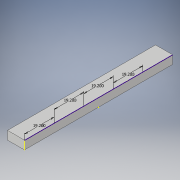
# Autodesk Inventor part: mars rover landscape part 2
Saved by Autodesk Inventor 2017 (Build 210142000, 142)
## iProperties
Created: 2017-09-13
Part Number: mars rover landscape part 2
Material: Generic
Document SubType Name: Modeling
Designer: 602199
Density: 1 g/cm^3
Appearance: Default
Author: 602199
Autodesk Inventor part; units mm, degrees
ref_plane "YZ Plane" through (0, 0, 0) normal (1, 0, 0) x (0, 1, 0)
ref_plane "XZ Plane" through (0, 0, 0) normal (0, 1, 0) x (-1, 0, 0)
ref_plane "XY Plane" through (0, 0, 0) normal (0, 0, 1) x (1, 0, 0)
sketch "Sketch1" plane through (0, 0, 0) normal (0, 1, 0) x (-1, 0, 0)
  line L0 (-139.7, 1219.2) -> (139.7, 1219.2)
  line L1 (139.7, 1219.2) -> (139.7, -1219.2)
  line L2 (139.7, -1219.2) -> (-139.7, -1219.2)
  line L3 (-139.7, -1219.2) -> (-139.7, 1219.2)
  line L4 (-139.7, 1219.2) -> (139.7, -1219.2) construction
  line L5 (139.7, 1219.2) -> (-139.7, -1219.2) construction
  point P0 (0, 0)
  dimension "d0" = 279.4
  dimension "d1" = 2438.4
  constraints: 12 end point, 2 midpoint, 2 parallel, 1 horizontal, 1 perpendicular
  measures "d0" distance of L1.end L2.end
  measures "d1" distance of L0.end L1.end
extrude "Extrusion1" add sketch "Sketch1" along normal blind 139.7
sketch "Sketch2" plane through (139.7, 0, 1219.2) normal (1, 0, 0) x (0, 0, -1)
  line L0 (0, 0) -> (0, 139.7) projected
  line L1 (0, 139.7) -> (487.68, 139.7)
  line L2 (0, 139.7) -> (2438.4, 139.7) projected
  line L3 (487.68, 139.7) -> (975.36, 139.7)
  line L4 (975.36, 139.7) -> (1463.04, 139.7)
  line L5 (1463.04, 139.7) -> (1950.72, 139.7)
  line L6 (1950.72, 139.7) -> (2438.4, 139.7)
  point P0 (1219.2, 0)
  dimension "d4" = 487.68
  dimension "d5" = 487.68
  dimension "d6" = 487.68
  dimension "d7" = 487.68
  constraints: 10 end point, 4 point on line, 1 collinear
  measures "d4" distance of L0.end L1.end
  measures "d5" distance of L1.end L3.end
  measures "d6" distance of L3.end L4.end
  measures "d7" distance of L4.end L5.end
body "Solid1"
